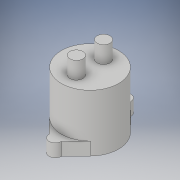
# Autodesk Inventor part: Precharge_Relay
Saved by Autodesk Inventor 2017 (Build 210142000, 142)
## iProperties
Created: 2017-02-06
Part Number: Precharge_Relay
Material: Generic
Document SubType Name: Modeling
Designer: plumbj
Density: 1 g/cm^3
Appearance: Default
Author: plumbj
Autodesk Inventor part; units mm, degrees
ref_plane "YZ Plane" through (0, 0, 0) normal (1, 0, 0) x (0, 1, 0)
ref_plane "XZ Plane" through (0, 0, 0) normal (0, 1, 0) x (-1, 0, 0)
ref_plane "XY Plane" through (0, 0, 0) normal (0, 0, 1) x (1, 0, 0)
sketch "Sketch1" plane through (0, 0, 0) normal (0, 1, 0) x (-1, 0, 0)
  circle A0 centre (0, 0) radius 28.067
  dimension "d0" = 56.134
  constraints: 1 centre point, 1 coincident
  measures "d0" diameter of A0
extrude "Extrusion1" add sketch "Sketch1" along normal blind 55.88
sketch "Sketch2" plane through (0, 55.88, 0) normal (0, 1, 0) x (1, 0, 0)
  circle A0 centre (0, -13.335) radius 6.35
  circle A1 centre (0, 13.335) radius 6.35
  point P0 (0, 0)
  dimension "d5" = 12.7
  dimension "d6" = 12.7
  constraints: 2 centre point
  measures "d5" diameter of A0
  measures "d6" diameter of A1
extrude "Extrusion2" add sketch "Sketch2" along normal blind 16.764
sketch "Sketch3" plane through (0, 0, 0) normal (0, -1, 0) x (1, 0, 0)
  circle A0 centre (0, 0) radius 28.067 projected
  circle A1 centre (0, 34.163) radius 6.096
  circle A2 centre (0, -34.163) radius 6.096
  line L0 (6.096, 34.163) -> (20.2372, 19.4477)
  line L1 (6.096, -34.163) -> (20.2372, -19.4477)
  line L2 (-6.096, 34.163) -> (-20.2372, 19.4477)
  line L3 (-6.096, -34.163) -> (-20.2372, -19.4477)
  constraints: 8 end point, 8 point on circle, 4 tangent, 2 centre point
extrude "Extrusion3" add sketch "Sketch3" against normal blind 12.7 contours A0 A1 L0 | A0 L2 A1 | A1
sketch "Sketch4" plane through (0, 0, 0) normal (0, -1, 0) x (1, 0, 0)
  circle A0 centre (0, 0) radius 28.067 projected
  circle A1 centre (0, -34.163) radius 6.096
  line L0 (6.096, -34.163) -> (20.2372, -19.4477)
  line L1 (-6.096, -34.163) -> (-20.2372, -19.4477)
  constraints: 4 end point, 4 point on circle, 2 tangent, 1 centre point
extrude "Extrusion4" add sketch "Sketch4" against normal blind 12.7
body "Solid1"
